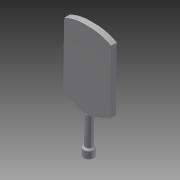
# Autodesk Inventor part: Pizza Bat
Saved by Autodesk Inventor 2015 (Build 190159000, 159)
## iProperties
Created: 2016-04-09
Part Number: Pizza Bat
Material: Generic
Document SubType Name: Modeling
Designer: tquinn
Density: 1 g/cm^3
Appearance: Default
Author: tquinn
Autodesk Inventor part; units mm, degrees
ref_plane "YZ Plane" through (0, 0, 0) normal (1, 0, 0) x (0, 1, 0)
ref_plane "XZ Plane" through (0, 0, 0) normal (0, 1, 0) x (-1, 0, 0)
ref_plane "XY Plane" through (0, 0, 0) normal (0, 0, 1) x (1, 0, 0)
sketch "Sketch1" plane through (0, 0, 0) normal (0, 0, 1) x (1, 0, 0)
  line L0 (63.363, 33.9802) -> (-9.3277, -37.5026) construction
  line L1 (-9.3277, -37.5026) -> (-80.8104, 35.188) construction
  line L2 (-80.8104, 35.188) -> (-8.1198, 106.6708) construction
  line L3 (-8.1198, 106.6708) -> (63.363, 33.9802) construction
  line L4 (-9.4479, -31.3777) -> (-7.3228, 95.6045)
  arc A0 (18.6765, 89.6068) -> (-19.9799, 93.6192) centre (-5.641, 43.5442) ccw
  line L5 (18.6765, 89.6068) -> (17.4956, 19.0471)
  line L6 (17.4956, 19.0471) -> (-1.6671, 11.2165)
  line L7 (-1.6671, 11.2165) -> (-5.0587, 9.8305)
  line L8 (-5.0587, 9.8305) -> (-5.4484, -21.9906)
  line L9 (-5.4484, -21.9906) -> (-3.8014, -23.6654)
  line L10 (-3.8014, -23.6654) -> (-3.932, -31.47)
  line L11 (-3.932, -31.47) -> (-9.4479, -31.3777)
  line L12 (-5.0587, 9.8305) -> (-8.7572, 9.8924)
  point P0 (0, 0)
  dimension "d1" = 127
  dimension "d2" = 101.9495
  constraints: 18 end point, 3 point on circle, 2 parallel, 2 perpendicular, 2 point on line, 1 centre point, 2 other
  measures "d1" distance of L4.start L4.end
  measures "d2" distance of L0.end L1.end
extrude "Extrusion2" add sketch "Sketch1" along normal mid plane 6.35 contours L4 A0 L5 L6 L7 L12
revolve "Revolution1" add sketch "Sketch1" angle 360 about axis through (-9.4479, -31.3777, 0) along (0.0167331, 0.99986, 0) contours L4 L12 L8 L9 L10 L11
mirror "Mirror2" about plane through (-7.3228, 95.6045, 0) normal (-0.99986, 0.0167331, 0) of "Extrusion2"
equation "\"d2\" = 0.802752 * d1"
body "Solid2"
